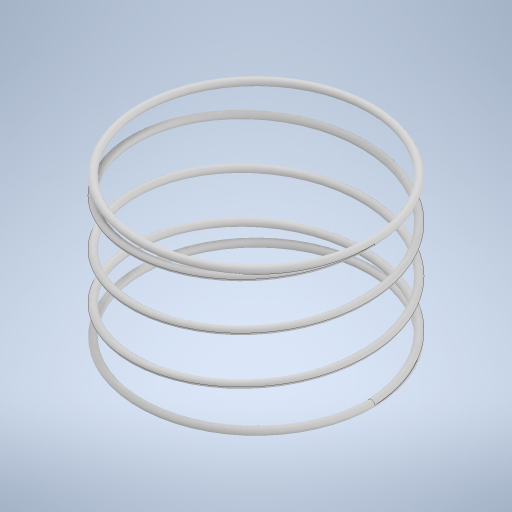
# Autodesk Inventor part: spring_V1
Saved by Autodesk Inventor 2023 (Build 270158000, 158)
## iProperties
Created: 2023-05-10
Part Number: spring_V1
Material: Generisch
Document SubType Name: Modeling
Designer: Mathi
Density: 1 g/cm^3
Appearance: Vorgabe
Author: Mathi
Autodesk Inventor part; units mm, degrees
ref_plane "YZ Plane" through (0, 0, 0) normal (1, 0, 0) x (0, 1, 0)
ref_plane "XZ Plane" through (0, 0, 0) normal (0, 1, 0) x (-1, 0, 0)
ref_plane "XY Plane" through (0, 0, 0) normal (0, 0, 1) x (1, 0, 0)
sketch "Skizze1" plane through (0, 0, 0) normal (0, 1, 0) x (-1, 0, 0)
  circle A0 centre (0, 0) radius 16.5
  dimension "d1" = 33
  constraints: 1 centre point, 1 coincident
  measures "d1" diameter of A0
sketch "Skizze2" plane through (0, 0, 0) normal (0, 0, 1) x (1, 0, 0)
  circle A0 centre (16.5, 0) radius 0.5
  line L0 (16.5, 0) -> (-16.5, 0) projected
  point P0 (0, 0)
  dimension "d2" = 1
  constraints: 1 centre point, 1 coincident
  measures "d2" diameter of A0
coil "Spirale1" sketch "Skizze2" operation add axis through (0, -10, 0) along (0, 1, 0) pitch 6.6667 turns 3 hand right
sketch "Skizze3" plane through (0, 0, 0) normal (0, 0, 1) x (1, 0, 0)
  circle A0 centre (16.5, 0) radius 0.5 projected
  circle A1 centre (16.5, 20) radius 0.5 projected
  line L0 (0, -4.7) -> (0, 24.7) projected
  point P0 (0, 0)
  point P1 (17, 0)
  point P2 (17, 20)
  constraints: 2 horizontal alignment
revolve "Umdrehung1" add sketch "Skizze3" angle 360 about axis through (0, -10, 0) along (0, 1, 0)
